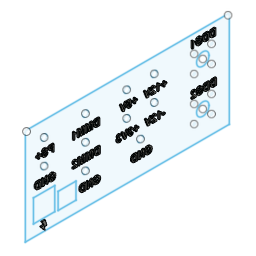
Schrift_Seitenteil_rechts (Autodesk Fusion 360 design; units mm, degrees)
Autodesk Fusion 360 part; units mm, degrees
(part 1 of 3)
sketch "Skizze1" plane through (-70, 0, 0) normal (-1, 0, 0) x (0, -1, 0)
  line L0 (-58.2934, 144.7089) -> (-56.3896, 144.7089)
  spline S0 degree 3 poles (-55.4941, 144.8148) (-55.624, 144.784) (-55.9182, 144.7143) (-56.2207, 144.7108) (-56.3896, 144.7089) knots 0 0 0 0 0.039934 0.090419 0.090419 0.090419 0.090419
  spline S1 degree 3 poles (-54.7832, 145.2147) (-54.8829, 145.1327) (-55.0958, 144.9574) (-55.3558, 144.8643) (-55.4941, 144.8148) knots 0 0 0 0 0.038436 0.082116 0.082116 0.082116 0.082116
  spline S2 degree 3 poles (-54.2466, 146.1) (-54.3131, 145.9292) (-54.4403, 145.6025) (-54.6724, 145.34) (-54.7832, 145.2147) knots 0 0 0 0 0.054482 0.104246 0.104246 0.104246 0.104246
  spline S3 degree 3 poles (-54.0928, 147.1664) (-54.0972, 146.9732) (-54.1056, 146.6113) (-54.2018, 146.2625) (-54.2466, 146.1) knots 0 0 0 0 0.057721 0.108107 0.108107 0.108107 0.108107
  spline S4 degree 3 poles (-54.2568, 148.3507) (-54.2091, 148.173) (-54.1049, 147.7854) (-54.097, 147.3838) (-54.0928, 147.1664) knots 0 0 0 0 0.055013 0.119956 0.119956 0.119956 0.119956
  spline S5 degree 3 poles (-54.7353, 149.1625) (-54.6361, 149.0437) (-54.4321, 148.7995) (-54.3163, 148.503) (-54.2568, 148.3507) knots 0 0 0 0 0.046108 0.094787 0.094787 0.094787 0.094787
  spline S6 degree 3 poles (-55.4907, 149.6239) (-55.3491, 149.5723) (-55.0663, 149.4692) (-54.8455, 149.2646) (-54.7353, 149.1625) knots 0 0 0 0 0.044725 0.089312 0.089312 0.089312 0.089312
  spline S7 degree 3 poles (-56.4443, 149.7196) (-56.2598, 149.7186) (-55.9386, 149.7169) (-55.6244, 149.6517) (-55.4907, 149.6239) knots 0 0 0 0 0.055167 0.096048 0.096048 0.096048 0.096048
  line L1 (-56.4443, 149.7196) -> (-58.2934, 149.7196)
  line L2 (-58.2934, 149.7196) -> (-58.2934, 144.7089)
  spline S8 degree 3 poles (-55.9966, 148.8241) (-56.101, 148.8379) (-56.3764, 148.8742) (-56.6545, 148.8728) (-56.8271, 148.872) knots 0 0 0 0 0.031565 0.083275 0.083275 0.083275 0.083275
  spline S9 degree 3 poles (-55.5283, 148.5883) (-55.5955, 148.642) (-55.7349, 148.7534) (-55.9073, 148.8) (-55.9966, 148.8241) knots 0 0 0 0 0.02553 0.052932 0.052932 0.052932 0.052932
  spline S10 degree 3 poles (-55.2412, 148.1029) (-55.2765, 148.1986) (-55.3427, 148.3782) (-55.4692, 148.5214) (-55.5283, 148.5883) knots 0 0 0 0 0.030297 0.056827 0.056827 0.056827 0.056827
  spline S11 degree 3 poles (-55.1387, 147.2108) (-55.1399, 147.3829) (-55.1421, 147.6843) (-55.2114, 147.9772) (-55.2412, 148.1029) knots 0 0 0 0 0.051419 0.090046 0.090046 0.090046 0.090046
  spline S12 degree 3 poles (-55.2412, 146.2931) (-55.2114, 146.4252) (-55.1433, 146.727) (-55.1403, 147.0367) (-55.1387, 147.2108) knots 0 0 0 0 0.040513 0.092572 0.092572 0.092572 0.092572
  spline S13 degree 3 poles (-55.5061, 145.8095) (-55.4529, 145.8719) (-55.3316, 146.0144) (-55.2737, 146.1929) (-55.2412, 146.2931) knots 0 0 0 0 0.024396 0.055616 0.055616 0.055616 0.055616
  spline S14 degree 3 poles (-55.9145, 145.601) (-55.8371, 145.624) (-55.688, 145.6684) (-55.5652, 145.7637) (-55.5061, 145.8095) knots 0 0 0 0 0.023993 0.046213 0.046213 0.046213 0.046213
  spline S15 degree 3 poles (-56.5264, 145.5531) (-56.4044, 145.5531) (-56.199, 145.553) (-55.9967, 145.5871) (-55.9145, 145.601) knots 0 0 0 0 0.036506 0.061461 0.061461 0.061461 0.061461
  line L3 (-56.5264, 145.5531) -> (-57.2817, 145.5531)
  line L4 (-57.2817, 145.5531) -> (-57.2817, 148.872)
  line L5 (-57.2817, 148.872) -> (-56.8271, 148.872)
  line L6 (-63.3486, 144.7089) -> (-61.4448, 144.7089)
  spline S16 degree 3 poles (-60.5493, 144.8148) (-60.6792, 144.784) (-60.9733, 144.7143) (-61.2759, 144.7108) (-61.4448, 144.7089) knots 0 0 0 0 0.039934 0.090419 0.090419 0.090419 0.090419
  spline S17 degree 3 poles (-59.8384, 145.2147) (-59.938, 145.1327) (-60.151, 144.9574) (-60.411, 144.8643) (-60.5493, 144.8148) knots 0 0 0 0 0.038436 0.082116 0.082116 0.082116 0.082116
  spline S18 degree 3 poles (-59.3017, 146.1) (-59.3683, 145.9292) (-59.4955, 145.6025) (-59.7276, 145.34) (-59.8384, 145.2147) knots 0 0 0 0 0.054482 0.104246 0.104246 0.104246 0.104246
  spline S19 degree 3 poles (-59.1479, 147.1664) (-59.1524, 146.9732) (-59.1608, 146.6113) (-59.2569, 146.2625) (-59.3017, 146.1) knots 0 0 0 0 0.057721 0.108107 0.108107 0.108107 0.108107
  spline S20 degree 3 poles (-59.312, 148.3507) (-59.2642, 148.173) (-59.1601, 147.7854) (-59.1522, 147.3838) (-59.1479, 147.1664) knots 0 0 0 0 0.055013 0.119956 0.119956 0.119956 0.119956
  spline S21 degree 3 poles (-59.7905, 149.1625) (-59.6913, 149.0437) (-59.4872, 148.7995) (-59.3715, 148.503) (-59.312, 148.3507) knots 0 0 0 0 0.046108 0.094787 0.094787 0.094787 0.094787
  spline S22 degree 3 poles (-60.5459, 149.6239) (-60.4043, 149.5723) (-60.1215, 149.4692) (-59.9007, 149.2646) (-59.7905, 149.1625) knots 0 0 0 0 0.044725 0.089312 0.089312 0.089312 0.089312
  spline S23 degree 3 poles (-61.4995, 149.7196) (-61.315, 149.7186) (-60.9938, 149.7169) (-60.6796, 149.6517) (-60.5459, 149.6239) knots 0 0 0 0 0.055167 0.096048 0.096048 0.096048 0.096048
  line L7 (-61.4995, 149.7196) -> (-63.3486, 149.7196)
  line L8 (-63.3486, 149.7196) -> (-63.3486, 144.7089)
  spline S24 degree 3 poles (-61.0517, 148.8241) (-61.1562, 148.8379) (-61.4316, 148.8742) (-61.7097, 148.8728) (-61.8823, 148.872) knots 0 0 0 0 0.031565 0.083275 0.083275 0.083275 0.083275
  spline S25 degree 3 poles (-60.5835, 148.5883) (-60.6507, 148.642) (-60.7901, 148.7534) (-60.9625, 148.8) (-61.0517, 148.8241) knots 0 0 0 0 0.02553 0.052932 0.052932 0.052932 0.052932
  spline S26 degree 3 poles (-60.2964, 148.1029) (-60.3317, 148.1986) (-60.3979, 148.3782) (-60.5244, 148.5214) (-60.5835, 148.5883) knots 0 0 0 0 0.030297 0.056827 0.056827 0.056827 0.056827
  spline S27 degree 3 poles (-60.1938, 147.2108) (-60.1951, 147.3829) (-60.1973, 147.6843) (-60.2666, 147.9772) (-60.2964, 148.1029) knots 0 0 0 0 0.051419 0.090046 0.090046 0.090046 0.090046
  spline S28 degree 3 poles (-60.2964, 146.2931) (-60.2666, 146.4252) (-60.1985, 146.727) (-60.1955, 147.0367) (-60.1938, 147.2108) knots 0 0 0 0 0.040513 0.092572 0.092572 0.092572 0.092572
  spline S29 degree 3 poles (-60.5613, 145.8095) (-60.5081, 145.8719) (-60.3868, 146.0144) (-60.3289, 146.1929) (-60.2964, 146.2931) knots 0 0 0 0 0.024396 0.055616 0.055616 0.055616 0.055616
  spline S30 degree 3 poles (-60.9697, 145.601) (-60.8923, 145.624) (-60.7432, 145.6684) (-60.6203, 145.7637) (-60.5613, 145.8095) knots 0 0 0 0 0.023993 0.046213 0.046213 0.046213 0.046213
  spline S31 degree 3 poles (-61.5815, 145.5531) (-61.4596, 145.5531) (-61.2542, 145.553) (-61.0519, 145.5871) (-60.9697, 145.601) knots 0 0 0 0 0.036506 0.061461 0.061461 0.061461 0.061461
  line L9 (-61.5815, 145.5531) -> (-62.3369, 145.5531)
  line L10 (-62.3369, 145.5531) -> (-62.3369, 148.872)
  line L11 (-62.3369, 148.872) -> (-61.8823, 148.872)
  spline S32 degree 3 poles (-51.4233, 144.62) (-51.7117, 144.6304) (-52.2389, 144.6493) (-52.6821, 144.9314) (-52.8828, 145.0592) knots 0 0 0 0 0.084711 0.154875 0.154875 0.154875 0.154875
  spline S33 degree 3 poles (-50.333, 144.8029) (-50.4955, 144.7496) (-50.8492, 144.6337) (-51.2218, 144.6248) (-51.4233, 144.62) knots 0 0 0 0 0.051012 0.111086 0.111086 0.111086 0.111086
  spline S34 degree 3 poles (-49.6562, 145.3617) (-49.7454, 145.2439) (-49.9268, 145.0044) (-50.1961, 144.8708) (-50.333, 144.8029) knots 0 0 0 0 0.043681 0.088839 0.088839 0.088839 0.088839
  spline S35 degree 3 poles (-49.417, 146.1683) (-49.4273, 146.0265) (-49.4482, 145.7402) (-49.5865, 145.4886) (-49.6562, 145.3617) knots 0 0 0 0 0.042126 0.085024 0.085024 0.085024 0.085024
  spline S36 degree 3 poles (-49.6169, 146.9664) (-49.5587, 146.8482) (-49.4348, 146.597) (-49.4232, 146.3167) (-49.417, 146.1683) knots 0 0 0 0 0.039093 0.083085 0.083085 0.083085 0.083085
  spline S37 degree 3 poles (-50.1706, 147.4757) (-50.0596, 147.4087) (-49.8405, 147.2764) (-49.6908, 147.0688) (-49.6169, 146.9664) knots 0 0 0 0 0.038473 0.075924 0.075924 0.075924 0.075924
  spline S38 degree 3 poles (-51.2627, 147.8363) (-51.0462, 147.7843) (-50.6719, 147.6945) (-50.3193, 147.5406) (-50.1706, 147.4757) knots 0 0 0 0 0.066618 0.115197 0.115197 0.115197 0.115197
  spline S39 degree 3 poles (-52.1924, 148.1713) (-52.0845, 148.1126) (-51.7928, 147.9541) (-51.4676, 147.8818) (-51.2627, 147.8363) knots 0 0 0 0 0.036685 0.099222 0.099222 0.099222 0.099222
  spline S40 degree 3 poles (-52.3428, 148.4755) (-52.3358, 148.4178) (-52.3215, 148.299) (-52.2362, 148.2147) (-52.1924, 148.1713) knots 0 0 0 0 0.016915 0.034837 0.034837 0.034837 0.034837
  spline S41 degree 3 poles (-52.1821, 148.7865) (-52.229, 148.7447) (-52.3222, 148.6614) (-52.3359, 148.5372) (-52.3428, 148.4755) knots 0 0 0 0 0.018159 0.036131 0.036131 0.036131 0.036131
  spline S42 degree 3 poles (-51.4917, 148.9677) (-51.6257, 148.9634) (-51.8706, 148.9557) (-52.0851, 148.8392) (-52.1821, 148.7865) knots 0 0 0 0 0.039567 0.07226 0.07226 0.07226 0.07226
  spline S43 degree 3 poles (-50.8508, 148.7985) (-50.9379, 148.8476) (-51.1357, 148.9594) (-51.3639, 148.9647) (-51.4917, 148.9677) knots 0 0 0 0 0.029564 0.067187 0.067187 0.067187 0.067187
  spline S44 degree 3 poles (-50.5723, 148.243) (-50.5959, 148.3591) (-50.639, 148.5704) (-50.785, 148.7276) (-50.8508, 148.7985) knots 0 0 0 0 0.034732 0.063204 0.063204 0.063204 0.063204
  line L12 (-50.5723, 148.243) -> (-49.5605, 148.2875)
  spline S45 degree 3 poles (-50.0613, 149.3915) (-49.9211, 149.2393) (-49.6335, 148.9268) (-49.5853, 148.5042) (-49.5605, 148.2875) knots 0 0 0 0 0.060438 0.124056 0.124056 0.124056 0.124056
  spline S46 degree 3 poles (-51.4814, 149.8051) (-51.1977, 149.7967) (-50.6859, 149.7816) (-50.2538, 149.5117) (-50.0613, 149.3915) knots 0 0 0 0 0.083316 0.150278 0.150278 0.150278 0.150278
  spline S47 degree 3 poles (-52.4675, 149.6307) (-52.3186, 149.6815) (-51.9992, 149.7904) (-51.6616, 149.8) (-51.4814, 149.8051) knots 0 0 0 0 0.046932 0.100643 0.100643 0.100643 0.100643
  spline S48 degree 3 poles (-53.093, 149.1232) (-53.0108, 149.2284) (-52.8414, 149.4453) (-52.5946, 149.5677) (-52.4675, 149.6307) knots 0 0 0 0 0.039537 0.081471 0.081471 0.081471 0.081471
  spline S49 degree 3 poles (-53.31, 148.4071) (-53.3006, 148.5332) (-53.2816, 148.788) (-53.1563, 149.0107) (-53.093, 149.1232) knots 0 0 0 0 0.037438 0.075643 0.075643 0.075643 0.075643
  spline S50 degree 3 poles (-52.8486, 147.3988) (-52.9832, 147.543) (-53.2492, 147.8281) (-53.2899, 148.2156) (-53.31, 148.4071) knots 0 0 0 0 0.057473 0.113615 0.113615 0.113615 0.113615
  spline S51 degree 3 poles (-51.707, 146.9032) (-51.9444, 146.9635) (-52.353, 147.0673) (-52.7023, 147.3009) (-52.8486, 147.3988) knots 0 0 0 0 0.072771 0.125248 0.125248 0.125248 0.125248
  spline S52 degree 3 poles (-50.897, 146.6845) (-50.9939, 146.7135) (-51.2619, 146.7939) (-51.5336, 146.8606) (-51.707, 146.9032) knots 0 0 0 0 0.030365 0.083919 0.083919 0.083919 0.083919
  spline S53 degree 3 poles (-50.5329, 146.4674) (-50.5789, 146.5092) (-50.6851, 146.6059) (-50.8202, 146.656) (-50.897, 146.6845) knots 0 0 0 0 0.018463 0.042727 0.042727 0.042727 0.042727
  spline S54 degree 3 poles (-50.4287, 146.1649) (-50.4326, 146.2214) (-50.4402, 146.3317) (-50.5025, 146.4229) (-50.5329, 146.4674) knots 0 0 0 0 0.016654 0.032515 0.032515 0.032515 0.032515
  spline S55 degree 3 poles (-50.6765, 145.6813) (-50.6043, 145.7509) (-50.4659, 145.8843) (-50.4407, 146.0742) (-50.4287, 146.1649) knots 0 0 0 0 0.02913 0.055793 0.055793 0.055793 0.055793
  spline S56 degree 3 poles (-51.4131, 145.4745) (-51.2662, 145.4785) (-51.0021, 145.4858) (-50.7766, 145.6212) (-50.6765, 145.6813) knots 0 0 0 0 0.043163 0.077652 0.077652 0.077652 0.077652
  spline S57 degree 3 poles (-52.1462, 145.7069) (-52.043, 145.6392) (-51.8212, 145.4937) (-51.5553, 145.4812) (-51.4131, 145.4745) knots 0 0 0 0 0.036365 0.078171 0.078171 0.078171 0.078171
  spline S58 degree 3 poles (-52.5068, 146.4349) (-52.4745, 146.2852) (-52.4153, 146.0111) (-52.2302, 145.8019) (-52.1462, 145.7069) knots 0 0 0 0 0.045039 0.082457 0.082457 0.082457 0.082457
  line L13 (-52.5068, 146.4349) -> (-53.4912, 146.3392)
  spline S59 degree 3 poles (-52.8828, 145.0592) (-53.0363, 145.2303) (-53.364, 145.5957) (-53.447, 146.0811) (-53.4912, 146.3392) knots 0 0 0 0 0.067573 0.144312 0.144312 0.144312 0.144312
  line L14 (-46.3203, 149.7401) -> (-47.0996, 149.7401)
  spline S60 degree 3 poles (-47.7046, 148.9386) (-47.5703, 149.0549) (-47.3111, 149.2791) (-47.1684, 149.5903) (-47.0996, 149.7401) knots 0 0 0 0 0.052597 0.101463 0.101463 0.101463 0.101463
  spline S61 degree 3 poles (-48.5215, 148.4721) (-48.388, 148.5266) (-48.0955, 148.6461) (-47.8423, 148.8356) (-47.7046, 148.9386) knots 0 0 0 0 0.043078 0.094413 0.094413 0.094413 0.094413
  line L15 (-48.5215, 148.4721) -> (-48.5215, 147.6005)
  spline S62 degree 3 poles (-47.2808, 148.3285) (-47.4653, 148.1747) (-47.8387, 147.8636) (-48.2922, 147.6888) (-48.5215, 147.6005) knots 0 0 0 0 0.071555 0.144721 0.144721 0.144721 0.144721
  line L16 (-47.2808, 148.3285) -> (-47.2808, 144.7089)
  line L17 (-47.2808, 144.7089) -> (-46.3203, 144.7089)
  line L18 (-46.3203, 144.7089) -> (-46.3203, 149.7401)
  line L19 (-63.8491, 113.2089) -> (-61.9453, 113.2089)
  spline S63 degree 3 poles (-61.0498, 113.3148) (-61.1797, 113.284) (-61.4739, 113.2143) (-61.7764, 113.2108) (-61.9453, 113.2089) knots 0 0 0 0 0.039934 0.090419 0.090419 0.090419 0.090419
  spline S64 degree 3 poles (-60.3389, 113.7147) (-60.4386, 113.6327) (-60.6515, 113.4574) (-60.9115, 113.3643) (-61.0498, 113.3148) knots 0 0 0 0 0.038436 0.082116 0.082116 0.082116 0.082116
  spline S65 degree 3 poles (-59.8023, 114.6) (-59.8688, 114.4292) (-59.996, 114.1025) (-60.2281, 113.84) (-60.3389, 113.7147) knots 0 0 0 0 0.054482 0.104246 0.104246 0.104246 0.104246
  spline S66 degree 3 poles (-59.6485, 115.6664) (-59.6529, 115.4732) (-59.6613, 115.1113) (-59.7575, 114.7625) (-59.8023, 114.6) knots 0 0 0 0 0.057721 0.108107 0.108107 0.108107 0.108107
  spline S67 degree 3 poles (-59.8125, 116.8507) (-59.7647, 116.673) (-59.6606, 116.2854) (-59.6527, 115.8838) (-59.6485, 115.6664) knots 0 0 0 0 0.055013 0.119956 0.119956 0.119956 0.119956
  spline S68 degree 3 poles (-60.291, 117.6625) (-60.1918, 117.5437) (-59.9878, 117.2995) (-59.872, 117.003) (-59.8125, 116.8507) knots 0 0 0 0 0.046108 0.094787 0.094787 0.094787 0.094787
  spline S69 degree 3 poles (-61.0464, 118.1239) (-60.9048, 118.0723) (-60.622, 117.9692) (-60.4012, 117.7646) (-60.291, 117.6625) knots 0 0 0 0 0.044725 0.089312 0.089312 0.089312 0.089312
  spline S70 degree 3 poles (-62, 118.2196) (-61.8155, 118.2186) (-61.4943, 118.2169) (-61.1801, 118.1517) (-61.0464, 118.1239) knots 0 0 0 0 0.055167 0.096048 0.096048 0.096048 0.096048
  line L20 (-62, 118.2196) -> (-63.8491, 118.2196)
  line L21 (-63.8491, 118.2196) -> (-63.8491, 113.2089)
  spline S71 degree 3 poles (-61.5523, 117.3241) (-61.6567, 117.3379) (-61.9321, 117.3742) (-62.2102, 117.3728) (-62.3828, 117.372) knots 0 0 0 0 0.031565 0.083275 0.083275 0.083275 0.083275
  spline S72 degree 3 poles (-61.084, 117.0883) (-61.1512, 117.142) (-61.2906, 117.2534) (-61.463, 117.3) (-61.5523, 117.3241) knots 0 0 0 0 0.02553 0.052932 0.052932 0.052932 0.052932
  spline S73 degree 3 poles (-60.7969, 116.6029) (-60.8322, 116.6986) (-60.8984, 116.8782) (-61.0249, 117.0214) (-61.084, 117.0883) knots 0 0 0 0 0.030297 0.056827 0.056827 0.056827 0.056827
  spline S74 degree 3 poles (-60.6944, 115.7108) (-60.6956, 115.8829) (-60.6978, 116.1843) (-60.7671, 116.4772) (-60.7969, 116.6029) knots 0 0 0 0 0.051419 0.090046 0.090046 0.090046 0.090046
  spline S75 degree 3 poles (-60.7969, 114.7931) (-60.7671, 114.9252) (-60.699, 115.227) (-60.696, 115.5367) (-60.6944, 115.7108) knots 0 0 0 0 0.040513 0.092572 0.092572 0.092572 0.092572
  spline S76 degree 3 poles (-61.0618, 114.3095) (-61.0086, 114.3719) (-60.8873, 114.5144) (-60.8294, 114.6929) (-60.7969, 114.7931) knots 0 0 0 0 0.024396 0.055616 0.055616 0.055616 0.055616
  spline S77 degree 3 poles (-61.4702, 114.101) (-61.3928, 114.124) (-61.2437, 114.1684) (-61.1209, 114.2637) (-61.0618, 114.3095) knots 0 0 0 0 0.023993 0.046213 0.046213 0.046213 0.046213
  spline S78 degree 3 poles (-62.082, 114.0531) (-61.9601, 114.0531) (-61.7547, 114.053) (-61.5524, 114.0871) (-61.4702, 114.101) knots 0 0 0 0 0.036506 0.061461 0.061461 0.061461 0.061461
  line L22 (-62.082, 114.0531) -> (-62.8374, 114.0531)
  line L23 (-62.8374, 114.0531) -> (-62.8374, 117.372)
  line L24 (-62.8374, 117.372) -> (-62.3828, 117.372)
  line L25 (-58.794, 113.2089) -> (-56.8902, 113.2089)
  spline S79 degree 3 poles (-55.9946, 113.3148) (-56.1245, 113.284) (-56.4187, 113.2143) (-56.7212, 113.2108) (-56.8902, 113.2089) knots 0 0 0 0 0.039934 0.090419 0.090419 0.090419 0.090419
  spline S80 degree 3 poles (-55.2837, 113.7147) (-55.3834, 113.6327) (-55.5963, 113.4574) (-55.8563, 113.3643) (-55.9946, 113.3148) knots 0 0 0 0 0.038436 0.082116 0.082116 0.082116 0.082116
  spline S81 degree 3 poles (-54.7471, 114.6) (-54.8136, 114.4292) (-54.9408, 114.1025) (-55.1729, 113.84) (-55.2837, 113.7147) knots 0 0 0 0 0.054482 0.104246 0.104246 0.104246 0.104246
  spline S82 degree 3 poles (-54.5933, 115.6664) (-54.5978, 115.4732) (-54.6061, 115.1113) (-54.7023, 114.7625) (-54.7471, 114.6) knots 0 0 0 0 0.057721 0.108107 0.108107 0.108107 0.108107
  spline S83 degree 3 poles (-54.7573, 116.8507) (-54.7096, 116.673) (-54.6054, 116.2854) (-54.5975, 115.8838) (-54.5933, 115.6664) knots 0 0 0 0 0.055013 0.119956 0.119956 0.119956 0.119956
  spline S84 degree 3 poles (-55.2359, 117.6625) (-55.1366, 117.5437) (-54.9326, 117.2995) (-54.8168, 117.003) (-54.7573, 116.8507) knots 0 0 0 0 0.046108 0.094787 0.094787 0.094787 0.094787
  spline S85 degree 3 poles (-55.9912, 118.1239) (-55.8496, 118.0723) (-55.5668, 117.9692) (-55.3461, 117.7646) (-55.2359, 117.6625) knots 0 0 0 0 0.044725 0.089312 0.089312 0.089312 0.089312
  spline S86 degree 3 poles (-56.9448, 118.2196) (-56.7604, 118.2186) (-56.4392, 118.2169) (-56.125, 118.1517) (-55.9912, 118.1239) knots 0 0 0 0 0.055167 0.096048 0.096048 0.096048 0.096048
  line L26 (-56.9448, 118.2196) -> (-58.794, 118.2196)
  line L27 (-58.794, 118.2196) -> (-58.794, 113.2089)
  spline S87 degree 3 poles (-56.4971, 117.3241) (-56.6015, 117.3379) (-56.877, 117.3742) (-57.155, 117.3728) (-57.3277, 117.372) knots 0 0 0 0 0.031565 0.083275 0.083275 0.083275 0.083275
  spline S88 degree 3 poles (-56.0288, 117.0883) (-56.096, 117.142) (-56.2354, 117.2534) (-56.4078, 117.3) (-56.4971, 117.3241) knots 0 0 0 0 0.02553 0.052932 0.052932 0.052932 0.052932
  spline S89 degree 3 poles (-55.7417, 116.6029) (-55.777, 116.6986) (-55.8432, 116.8782) (-55.9698, 117.0214) (-56.0288, 117.0883) knots 0 0 0 0 0.030297 0.056827 0.056827 0.056827 0.056827
  spline S90 degree 3 poles (-55.6392, 115.7108) (-55.6404, 115.8829) (-55.6426, 116.1843) (-55.712, 116.4772) (-55.7417, 116.6029) knots 0 0 0 0 0.051419 0.090046 0.090046 0.090046 0.090046
  spline S91 degree 3 poles (-55.7417, 114.7931) (-55.7119, 114.9252) (-55.6439, 115.227) (-55.6409, 115.5367) (-55.6392, 115.7108) knots 0 0 0 0 0.040513 0.092572 0.092572 0.092572 0.092572
  spline S92 degree 3 poles (-56.0066, 114.3095) (-55.9534, 114.3719) (-55.8321, 114.5144) (-55.7742, 114.6929) (-55.7417, 114.7931) knots 0 0 0 0 0.024396 0.055616 0.055616 0.055616 0.055616
  spline S93 degree 3 poles (-56.4151, 114.101) (-56.3376, 114.124) (-56.1885, 114.1684) (-56.0657, 114.2637) (-56.0066, 114.3095) knots 0 0 0 0 0.023993 0.046213 0.046213 0.046213 0.046213
  spline S94 degree 3 poles (-57.0269, 114.0531) (-56.9049, 114.0531) (-56.6995, 114.053) (-56.4972, 114.0871) (-56.4151, 114.101) knots 0 0 0 0 0.036506 0.061461 0.061461 0.061461 0.061461
  line L28 (-57.0269, 114.0531) -> (-57.7822, 114.0531)
  line L29 (-57.7822, 114.0531) -> (-57.7822, 117.372)
  line L30 (-57.7822, 117.372) -> (-57.3277, 117.372)
  spline S95 degree 3 poles (-51.9238, 113.12) (-52.2122, 113.1304) (-52.7395, 113.1493) (-53.1826, 113.4314) (-53.3833, 113.5592) knots 0 0 0 0 0.084711 0.154875 0.154875 0.154875 0.154875
  spline S96 degree 3 poles (-50.8335, 113.3029) (-50.996, 113.2496) (-51.3497, 113.1337) (-51.7223, 113.1248) (-51.9238, 113.12) knots 0 0 0 0 0.051012 0.111086 0.111086 0.111086 0.111086
  spline S97 degree 3 poles (-50.1568, 113.8617) (-50.2459, 113.7439) (-50.4273, 113.5044) (-50.6966, 113.3708) (-50.8335, 113.3029) knots 0 0 0 0 0.043681 0.088839 0.088839 0.088839 0.088839
  spline S98 degree 3 poles (-49.9175, 114.6683) (-49.9278, 114.5265) (-49.9487, 114.2402) (-50.087, 113.9886) (-50.1568, 113.8617) knots 0 0 0 0 0.042126 0.085024 0.085024 0.085024 0.085024
  spline S99 degree 3 poles (-50.1174, 115.4664) (-50.0592, 115.3482) (-49.9354, 115.097) (-49.9237, 114.8167) (-49.9175, 114.6683) knots 0 0 0 0 0.039093 0.083085 0.083085 0.083085 0.083085
  spline S100 degree 3 poles (-50.6712, 115.9757) (-50.5601, 115.9087) (-50.341, 115.7764) (-50.1913, 115.5688) (-50.1174, 115.4664) knots 0 0 0 0 0.038473 0.075924 0.075924 0.075924 0.075924
  spline S101 degree 3 poles (-51.7632, 116.3363) (-51.5467, 116.2843) (-51.1724, 116.1945) (-50.8198, 116.0406) (-50.6712, 115.9757) knots 0 0 0 0 0.066618 0.115197 0.115197 0.115197 0.115197
  spline S102 degree 3 poles (-52.6929, 116.6713) (-52.585, 116.6126) (-52.2933, 116.4541) (-51.9682, 116.3818) (-51.7632, 116.3363) knots 0 0 0 0 0.036685 0.099222 0.099222 0.099222 0.099222
  spline S103 degree 3 poles (-52.8433, 116.9755) (-52.8363, 116.9178) (-52.822, 116.799) (-52.7367, 116.7147) (-52.6929, 116.6713) knots 0 0 0 0 0.016915 0.034837 0.034837 0.034837 0.034837
  spline S104 degree 3 poles (-52.6826, 117.2865) (-52.7295, 117.2447) (-52.8227, 117.1614) (-52.8364, 117.0372) (-52.8433, 116.9755) knots 0 0 0 0 0.018159 0.036131 0.036131 0.036131 0.036131
  spline S105 degree 3 poles (-51.9922, 117.4677) (-52.1263, 117.4634) (-52.3711, 117.4557) (-52.5856, 117.3392) (-52.6826, 117.2865) knots 0 0 0 0 0.039567 0.07226 0.07226 0.07226 0.07226
  spline S106 degree 3 poles (-51.3513, 117.2985) (-51.4384, 117.3476) (-51.6362, 117.4594) (-51.8644, 117.4647) (-51.9922, 117.4677) knots 0 0 0 0 0.029564 0.067187 0.067187 0.067187 0.067187
  spline S107 degree 3 poles (-51.0728, 116.743) (-51.0964, 116.8591) (-51.1395, 117.0704) (-51.2856, 117.2276) (-51.3513, 117.2985) knots 0 0 0 0 0.034732 0.063204 0.063204 0.063204 0.063204
  line L31 (-51.0728, 116.743) -> (-50.061, 116.7875)
  spline S108 degree 3 poles (-50.5618, 117.8915) (-50.4216, 117.7393) (-50.134, 117.4268) (-50.0858, 117.0042) (-50.061, 116.7875) knots 0 0 0 0 0.060438 0.124056 0.124056 0.124056 0.124056
  spline S109 degree 3 poles (-51.9819, 118.3051) (-51.6982, 118.2967) (-51.1864, 118.2816) (-50.7543, 118.0117) (-50.5618, 117.8915) knots 0 0 0 0 0.083316 0.150278 0.150278 0.150278 0.150278
  spline S110 degree 3 poles (-52.968, 118.1307) (-52.8191, 118.1815) (-52.4997, 118.2904) (-52.1621, 118.3) (-51.9819, 118.3051) knots 0 0 0 0 0.046932 0.100643 0.100643 0.100643 0.100643
  spline S111 degree 3 poles (-53.5935, 117.6232) (-53.5113, 117.7284) (-53.3419, 117.9453) (-53.0951, 118.0677) (-52.968, 118.1307) knots 0 0 0 0 0.039537 0.081471 0.081471 0.081471 0.081471
  spline S112 degree 3 poles (-53.8106, 116.9071) (-53.8012, 117.0332) (-53.7822, 117.288) (-53.6568, 117.5107) (-53.5935, 117.6232) knots 0 0 0 0 0.037438 0.075643 0.075643 0.075643 0.075643
  spline S113 degree 3 poles (-53.3491, 115.8988) (-53.4837, 116.043) (-53.7497, 116.3281) (-53.7904, 116.7156) (-53.8106, 116.9071) knots 0 0 0 0 0.057473 0.113615 0.113615 0.113615 0.113615
  spline S114 degree 3 poles (-52.2075, 115.4032) (-52.4449, 115.4635) (-52.8535, 115.5673) (-53.2028, 115.8009) (-53.3491, 115.8988) knots 0 0 0 0 0.072771 0.125248 0.125248 0.125248 0.125248
  spline S115 degree 3 poles (-51.3975, 115.1845) (-51.4944, 115.2135) (-51.7624, 115.2939) (-52.0341, 115.3606) (-52.2075, 115.4032) knots 0 0 0 0 0.030365 0.083919 0.083919 0.083919 0.083919
  spline S116 degree 3 poles (-51.0335, 114.9674) (-51.0794, 115.0092) (-51.1856, 115.1059) (-51.3207, 115.156) (-51.3975, 115.1845) knots 0 0 0 0 0.018463 0.042727 0.042727 0.042727 0.042727
  spline S117 degree 3 poles (-50.9292, 114.6649) (-50.9331, 114.7214) (-50.9407, 114.8317) (-51.0031, 114.9229) (-51.0335, 114.9674) knots 0 0 0 0 0.016654 0.032515 0.032515 0.032515 0.032515
  spline S118 degree 3 poles (-51.177, 114.1813) (-51.1048, 114.2509) (-50.9664, 114.3843) (-50.9412, 114.5742) (-50.9292, 114.6649) knots 0 0 0 0 0.02913 0.055793 0.055793 0.055793 0.055793
  spline S119 degree 3 poles (-51.9136, 113.9745) (-51.7668, 113.9785) (-51.5026, 113.9858) (-51.2772, 114.1212) (-51.177, 114.1813) knots 0 0 0 0 0.043163 0.077652 0.077652 0.077652 0.077652
  spline S120 degree 3 poles (-52.6467, 114.2069) (-52.5435, 114.1392) (-52.3217, 113.9937) (-52.0558, 113.9812) (-51.9136, 113.9745) knots 0 0 0 0 0.036365 0.078171 0.078171 0.078171 0.078171
  spline S121 degree 3 poles (-53.0073, 114.9349) (-52.975, 114.7852) (-52.9158, 114.5111) (-52.7307, 114.3019) (-52.6467, 114.2069) knots 0 0 0 0 0.045039 0.082457 0.082457 0.082457 0.082457
  line L32 (-53.0073, 114.9349) -> (-53.9917, 114.8392)
  spline S122 degree 3 poles (-53.3833, 113.5592) (-53.5368, 113.7303) (-53.8645, 114.0957) (-53.9476, 114.5811) (-53.9917, 114.8392) knots 0 0 0 0 0.067573 0.144312 0.144312 0.144312 0.144312
  spline S123 degree 3 poles (-47.7454, 114.3676) (-47.7832, 114.3235) (-47.8553, 114.2394) (-47.914, 114.1456) (-47.9419, 114.101) knots 0 0 0 0 0.017402 0.033163 0.033163 0.033163 0.033163
  spline S124 degree 3 poles (-47.1694, 114.9213) (-47.2947, 114.8071) (-47.4916, 114.6277) (-47.6776, 114.437) (-47.7454, 114.3676) knots 0 0 0 0 0.050814 0.079907 0.079907 0.079907 0.079907
  spline S125 degree 3 poles (-46.5405, 115.5604) (-46.6207, 115.4689) (-46.8179, 115.2437) (-47.0385, 115.0414) (-47.1694, 114.9213) knots 0 0 0 0 0.036482 0.089726 0.089726 0.089726 0.089726
  spline S126 degree 3 poles (-46.156, 116.2013) (-46.2049, 116.0949) (-46.3096, 115.8673) (-46.4603, 115.6671) (-46.5405, 115.5604) knots 0 0 0 0 0.035023 0.074928 0.074928 0.074928 0.074928
  spline S127 degree 3 poles (-46.0347, 116.8456) (-46.0396, 116.7345) (-46.0493, 116.5139) (-46.1206, 116.305) (-46.156, 116.2013) knots 0 0 0 0 0.033165 0.06586 0.06586 0.06586 0.06586
  spline S128 degree 3 poles (-46.4585, 117.8402) (-46.3349, 117.6982) (-46.0862, 117.4126) (-46.0519, 117.0353) (-46.0347, 116.8456) knots 0 0 0 0 0.054981 0.110602 0.110602 0.110602 0.110602
  spline S129 degree 3 poles (-47.624, 118.2401) (-47.3956, 118.2284) (-46.9672, 118.2064) (-46.6204, 117.9567) (-46.4585, 117.8402) knots 0 0 0 0 0.066974 0.125562 0.125562 0.125562 0.125562
  spline S130 degree 3 poles (-48.752, 117.8949) (-48.5873, 117.9955) (-48.2416, 118.2068) (-47.8363, 118.2287) (-47.624, 118.2401) knots 0 0 0 0 0.056979 0.119613 0.119613 0.119613 0.119613
  spline S131 degree 3 poles (-49.2886, 116.7567) (-49.2532, 116.9954) (-49.1885, 117.4315) (-48.888, 117.7505) (-48.752, 117.8949) knots 0 0 0 0 0.070363 0.128535 0.128535 0.128535 0.128535
  line L33 (-49.2886, 116.7567) -> (-48.3316, 116.661)
  spline S132 degree 3 poles (-48.1265, 117.2626) (-48.1797, 117.1847) (-48.303, 117.0043) (-48.3212, 116.7854) (-48.3316, 116.661) knots 0 0 0 0 0.027875 0.064515 0.064515 0.064515 0.064515
  spline S133 degree 3 poles (-47.648, 117.4437) (-47.7415, 117.4377) (-47.9201, 117.4263) (-48.0599, 117.3154) (-48.1265, 117.2626) knots 0 0 0 0 0.027379 0.052265 0.052265 0.052265 0.052265
  spline S134 degree 3 poles (-47.1712, 117.2711) (-47.237, 117.3214) (-47.3772, 117.4286) (-47.5541, 117.4385) (-47.648, 117.4437) knots 0 0 0 0 0.024288 0.051759 0.051759 0.051759 0.051759
  spline S135 degree 3 poles (-46.9985, 116.7772) (-47.0033, 116.8755) (-47.012, 117.058) (-47.1209, 117.2038) (-47.1712, 117.2711) knots 0 0 0 0 0.028738 0.053388 0.053388 0.053388 0.053388
  spline S136 degree 3 poles (-47.1968, 116.1893) (-47.139, 116.2852) (-47.0295, 116.4669) (-47.0085, 116.6777) (-46.9985, 116.7772) knots 0 0 0 0 0.033093 0.062734 0.062734 0.062734 0.062734
  spline S137 degree 3 poles (-47.9932, 115.369) (-47.8138, 115.5337) (-47.5325, 115.7921) (-47.2861, 116.0836) (-47.1968, 116.1893) knots 0 0 0 0 0.072938 0.114424 0.114424 0.114424 0.114424
  spline S138 degree 3 poles (-49.0733, 114.1676) (-48.942, 114.347) (-48.6228, 114.7834) (-48.2265, 115.152) (-47.9932, 115.369) knots 0 0 0 0 0.066554 0.16187 0.16187 0.16187 0.16187
  spline S139 degree 3 poles (-49.4014, 113.2089) (-49.3736, 113.376) (-49.3174, 113.7138) (-49.1552, 114.0153) (-49.0733, 114.1676) knots 0 0 0 0 0.050461 0.101951 0.101951 0.101951 0.101951
  line L34 (-49.4014, 113.2089) -> (-46.0347, 113.2089)
  line L35 (-46.0347, 113.2089) -> (-46.0347, 114.101)
  line L36 (-46.0347, 114.101) -> (-47.9419, 114.101)
  line L37 (4.1011, 130.5054) -> (5.8956, 135.5162)
  line L38 (5.8956, 135.5162) -> (4.8223, 135.5162)
  line L39 (4.8223, 135.5162) -> (3.5953, 131.8077)
  line L40 (3.5953, 131.8077) -> (2.3272, 135.5162)
  line L41 (2.3272, 135.5162) -> (1.23, 135.5162)
  line L42 (1.23, 135.5162) -> (3.0211, 130.5054)
  line L43 (3.0211, 130.5054) -> (4.1011, 130.5054)
  spline S140 degree 3 poles (-0.6943, 130.42) (-0.9106, 130.4321) (-1.3222, 130.455) (-1.6637, 130.684) (-1.8256, 130.7926) knots 0 0 0 0 0.063661 0.121078 0.121078 0.121078 0.121078
  spline S141 degree 3 poles (0.6627, 131.0831) (0.4818, 130.8897) (0.1142, 130.4968) (-0.422, 130.4459) (-0.6943, 130.42) knots 0 0 0 0 0.076677 0.155765 0.155765 0.155765 0.155765
  spline S142 degree 3 poles (1.0216, 132.1871) (1.007, 131.987) (0.9781, 131.5894) (0.7673, 131.2511) (0.6627, 131.0831) knots 0 0 0 0 0.059216 0.117652 0.117652 0.117652 0.117652
  spline S143 degree 3 poles (0.5772, 133.3936) (0.7068, 133.2226) (0.9766, 132.8663) (1.0062, 132.4194) (1.0216, 132.1871) knots 0 0 0 0 0.06295 0.13111 0.13111 0.13111 0.13111
  spline S144 degree 3 poles (-0.5063, 133.8585) (-0.3012, 133.839) (0.1096, 133.7999) (0.4212, 133.5292) (0.5772, 133.3936) knots 0 0 0 0 0.060178 0.120563 0.120563 0.120563 0.120563
  spline S145 degree 3 poles (-1.1625, 133.6978) (-1.0559, 133.7447) (-0.8465, 133.8367) (-0.6183, 133.8513) (-0.5063, 133.8585) knots 0 0 0 0 0.034634 0.068031 0.068031 0.068031 0.068031
  line L44 (-1.1625, 133.6978) -> (-1.0121, 134.5489)
  line L45 (-1.0121, 134.5489) -> (0.7994, 134.5489)
  line L46 (0.7994, 134.5489) -> (0.7994, 135.4478)
  line L47 (0.7994, 135.4478) -> (-1.7402, 135.4478)
  line L48 (-1.7402, 135.4478) -> (-2.2324, 132.8399)
  line L49 (-2.2324, 132.8399) -> (-1.4531, 132.7271)
  spline S146 degree 3 poles (-0.7114, 133.0929) (-0.8481, 133.0748) (-1.1356, 133.0369) (-1.3438, 132.8337) (-1.4531, 132.7271) knots 0 0 0 0 0.040273 0.0847 0.0847 0.0847 0.0847
  spline S147 degree 3 poles (-0.173, 132.8621) (-0.2482, 132.9294) (-0.4015, 133.0666) (-0.6067, 133.084) (-0.7114, 133.0929) knots 0 0 0 0 0.029423 0.060008 0.060008 0.060008 0.060008
  spline S148 degree 3 poles (0.0338, 132.17) (0.0296, 132.3088) (0.022, 132.5592) (-0.1129, 132.7687) (-0.173, 132.8621) knots 0 0 0 0 0.040704 0.073449 0.073449 0.073449 0.073449
  spline S149 degree 3 poles (-0.1747, 131.4334) (-0.1141, 131.533) (0.0228, 131.7579) (0.0299, 132.0225) (0.0338, 132.17) knots 0 0 0 0 0.034394 0.077732 0.077732 0.077732 0.077732
  spline S150 degree 3 poles (-0.684, 131.189) (-0.587, 131.2) (-0.3891, 131.2223) (-0.2471, 131.3622) (-0.1747, 131.4334) knots 0 0 0 0 0.028435 0.057968 0.057968 0.057968 0.057968
  spline S151 degree 3 poles (-1.1489, 131.3787) (-1.0797, 131.3234) (-0.9433, 131.2143) (-0.7696, 131.1974) (-0.684, 131.189) knots 0 0 0 0 0.025952 0.051182 0.051182 0.051182 0.051182
  spline S152 degree 3 poles (-1.3915, 131.8931) (-1.3728, 131.7921) (-1.337, 131.5989) (-1.2096, 131.4499) (-1.1489, 131.3787) knots 0 0 0 0 0.030207 0.057777 0.057777 0.057777 0.057777
  line L50 (-1.3915, 131.8931) -> (-2.3486, 131.794)
  spline S153 degree 3 poles (-1.8256, 130.7926) (-1.9571, 130.9302) (-2.2276, 131.2131) (-2.3075, 131.5969) (-2.3486, 131.794) knots 0 0 0 0 0.055929 0.115014 0.115014 0.115014 0.115014
  line L51 (-4.2695, 131.2266) -> (-4.2695, 132.5289)
  line L52 (-4.2695, 132.5289) -> (-2.9535, 132.5289)
  line L53 (-2.9535, 132.5289) -> (-2.9535, 133.4278)
  line L54 (-2.9535, 133.4278) -> (-4.2695, 133.4278)
  line L55 (-4.2695, 133.4278) -> (-4.2695, 134.7301)
  line L56 (-4.2695, 134.7301) -> (-5.1445, 134.7301)
  line L57 (-5.1445, 134.7301) -> (-5.1445, 133.4278)
  line L58 (-5.1445, 133.4278) -> (-6.457, 133.4278)
  line L59 (-6.457, 133.4278) -> (-6.457, 132.5289)
  line L60 (-6.457, 132.5289) -> (-5.1445, 132.5289)
  line L61 (-5.1445, 132.5289) -> (-5.1445, 131.2266)
  line L62 (-5.1445, 131.2266) -> (-4.2695, 131.2266)
  line L63 (-13.3696, 130.42) -> (-11.5752, 135.4307)
  line L64 (-11.5752, 135.4307) -> (-12.6484, 135.4307)
  line L65 (-12.6484, 135.4307) -> (-13.8755, 131.7222)
  line L66 (-13.8755, 131.7222) -> (-15.1436, 135.4307)
  line L67 (-15.1436, 135.4307) -> (-16.2407, 135.4307)
  line L68 (-16.2407, 135.4307) -> (-14.4497, 130.42)
  line L69 (-14.4497, 130.42) -> (-13.3696, 130.42)
  spline S154 degree 3 poles (-18.3001, 131.5787) (-18.3379, 131.5346) (-18.41, 131.4505) (-18.4687, 131.3567) (-18.4966, 131.3121) knots 0 0 0 0 0.017402 0.033163 0.033163 0.033163 0.033163
  spline S155 degree 3 poles (-17.7241, 132.1324) (-17.8494, 132.0183) (-18.0463, 131.8388) (-18.2323, 131.6481) (-18.3001, 131.5787) knots 0 0 0 0 0.050814 0.079907 0.079907 0.079907 0.079907
  spline S156 degree 3 poles (-17.0952, 132.7716) (-17.1754, 132.68) (-17.3726, 132.4549) (-17.5932, 132.2525) (-17.7241, 132.1324) knots 0 0 0 0 0.036482 0.089726 0.089726 0.089726 0.089726
  spline S157 degree 3 poles (-16.7107, 133.4124) (-16.7596, 133.306) (-16.8643, 133.0785) (-17.015, 132.8782) (-17.0952, 132.7716) knots 0 0 0 0 0.035023 0.074928 0.074928 0.074928 0.074928
  spline S158 degree 3 poles (-16.5894, 134.0567) (-16.5943, 133.9456) (-16.604, 133.7251) (-16.6753, 133.5162) (-16.7107, 133.4124) knots 0 0 0 0 0.033165 0.06586 0.06586 0.06586 0.06586
  spline S159 degree 3 poles (-17.0132, 135.0513) (-16.8896, 134.9094) (-16.6409, 134.6237) (-16.6066, 134.2465) (-16.5894, 134.0567) knots 0 0 0 0 0.054981 0.110602 0.110602 0.110602 0.110602
  spline S160 degree 3 poles (-18.1787, 135.4513) (-17.9503, 135.4395) (-17.5219, 135.4175) (-17.175, 135.1678) (-17.0132, 135.0513) knots 0 0 0 0 0.066973 0.125562 0.125562 0.125562 0.125562
  spline S161 degree 3 poles (-19.3067, 135.106) (-19.142, 135.2067) (-18.7963, 135.4179) (-18.391, 135.4398) (-18.1787, 135.4513) knots 0 0 0 0 0.056979 0.119613 0.119613 0.119613 0.119613
  spline S162 degree 3 poles (-19.8433, 133.9679) (-19.8079, 134.2065) (-19.7432, 134.6426) (-19.4427, 134.9616) (-19.3067, 135.106) knots 0 0 0 0 0.070363 0.128535 0.128535 0.128535 0.128535
  line L70 (-19.8433, 133.9679) -> (-18.8862, 133.8721)
  spline S163 degree 3 poles (-18.6812, 134.4737) (-18.7344, 134.3958) (-18.8576, 134.2155) (-18.8759, 133.9965) (-18.8862, 133.8721) knots 0 0 0 0 0.027875 0.064515 0.064515 0.064515 0.064515
  spline S164 degree 3 poles (-18.2026, 134.6549) (-18.2962, 134.6489) (-18.4748, 134.6374) (-18.6146, 134.5265) (-18.6812, 134.4737) knots 0 0 0 0 0.027379 0.052265 0.052265 0.052265 0.052265
  spline S165 degree 3 poles (-17.7258, 134.4823) (-17.7917, 134.5325) (-17.9319, 134.6397) (-18.1088, 134.6496) (-18.2026, 134.6549) knots 0 0 0 0 0.024288 0.051759 0.051759 0.051759 0.051759
  spline S166 degree 3 poles (-17.5532, 133.9884) (-17.5579, 134.0866) (-17.5667, 134.2692) (-17.6756, 134.4149) (-17.7258, 134.4823) knots 0 0 0 0 0.028738 0.053388 0.053388 0.053388 0.053388
  spline S167 degree 3 poles (-17.7515, 133.4005) (-17.6937, 133.4963) (-17.5842, 133.678) (-17.5632, 133.8888) (-17.5532, 133.9884) knots 0 0 0 0 0.033093 0.062734 0.062734 0.062734 0.062734
  spline S168 degree 3 poles (-18.5479, 132.5802) (-18.3685, 132.7449) (-18.0872, 133.0032) (-17.8408, 133.2948) (-17.7515, 133.4005) knots 0 0 0 0 0.072938 0.114424 0.114424 0.114424 0.114424
  spline S169 degree 3 poles (-19.6279, 131.3787) (-19.4967, 131.5582) (-19.1775, 131.9945) (-18.7812, 132.3631) (-18.5479, 132.5802) knots 0 0 0 0 0.066554 0.16187 0.16187 0.16187 0.16187
  spline S170 degree 3 poles (-19.9561, 130.42) (-19.9283, 130.5872) (-19.8721, 130.9249) (-19.7099, 131.2264) (-19.6279, 131.3787) knots 0 0 0 0 0.050461 0.101951 0.101951 0.101951 0.101951
  line L71 (-19.9561, 130.42) -> (-16.5894, 130.42)
  line L72 (-16.5894, 130.42) -> (-16.5894, 131.3121)
  line L73 (-16.5894, 131.3121) -> (-18.4966, 131.3121)
  line L74 (-21.2686, 135.4513) -> (-22.0479, 135.4513)
  spline S171 degree 3 poles (-22.6528, 134.6497) (-22.5185, 134.766) (-22.2594, 134.9903) (-22.1166, 135.3014) (-22.0479, 135.4513) knots 0 0 0 0 0.052597 0.101463 0.101463 0.101463 0.101463
  spline S172 degree 3 poles (-23.4697, 134.1832) (-23.3363, 134.2377) (-23.0438, 134.3572) (-22.7905, 134.5467) (-22.6528, 134.6497) knots 0 0 0 0 0.043078 0.094413 0.094413 0.094413 0.094413
  line L75 (-23.4697, 134.1832) -> (-23.4697, 133.3116)
  spline S173 degree 3 poles (-22.229, 134.0396) (-22.4136, 133.8858) (-22.7869, 133.5747) (-23.2405, 133.4) (-23.4697, 133.3116) knots 0 0 0 0 0.071555 0.144721 0.144721 0.144721 0.144721
  line L76 (-22.229, 134.0396) -> (-22.229, 130.42)
  line L77 (-22.229, 130.42) -> (-21.2686, 130.42)
  line L78 (-21.2686, 130.42) -> (-21.2686, 135.4513)
  line L79 (-25.6333, 131.1412) -> (-25.6333, 132.4434)
  line L80 (-25.6333, 132.4434) -> (-24.3174, 132.4434)
  line L81 (-24.3174, 132.4434) -> (-24.3174, 133.3424)
  line L82 (-24.3174, 133.3424) -> (-25.6333, 133.3424)
  line L83 (-25.6333, 133.3424) -> (-25.6333, 134.6446)
  line L84 (-25.6333, 134.6446) -> (-26.5083, 134.6446)
  line L85 (-26.5083, 134.6446) -> (-26.5083, 133.3424)
  line L86 (-26.5083, 133.3424) -> (-27.8208, 133.3424)
  line L87 (-27.8208, 133.3424) -> (-27.8208, 132.4434)
  line L88 (-27.8208, 132.4434) -> (-26.5083, 132.4434)
  line L89 (-26.5083, 132.4434) -> (-26.5083, 131.1412)
  line L90 (-26.5083, 131.1412) -> (-25.6333, 131.1412)
  line L91 (-24.798, 113.7564) -> (-24.798, 114.7169)
  line L92 (-24.798, 114.7169) -> (-26.6847, 114.7169)
  line L93 (-26.6847, 114.7169) -> (-26.6847, 113.7564)
  line L94 (-26.6847, 113.7564) -> (-24.798, 113.7564)
  line L95 (-21.9919, 117.4513) -> (-22.7712, 117.4513)
  spline S174 degree 3 poles (-23.3762, 116.6497) (-23.2418, 116.766) (-22.9827, 116.9903) (-22.8399, 117.3014) (-22.7712, 117.4513) knots 0 0 0 0 0.052597 0.101463 0.101463 0.101463 0.101463
  spline S175 degree 3 poles (-24.193, 116.1832) (-24.0596, 116.2377) (-23.7671, 116.3572) (-23.5138, 116.5467) (-23.3762, 116.6497) knots 0 0 0 0 0.043078 0.094413 0.094413 0.094413 0.094413
  line L96 (-24.193, 116.1832) -> (-24.193, 115.3116)
  spline S176 degree 3 poles (-22.9523, 116.0396) (-23.1369, 115.8858) (-23.5102, 115.5747) (-23.9638, 115.4) (-24.193, 115.3116) knots 0 0 0 0 0.071555 0.144721 0.144721 0.144721 0.144721
  line L97 (-22.9523, 116.0396) -> (-22.9523, 112.42)
  line L98 (-22.9523, 112.42) -> (-21.9919, 112.42)
  line L99 (-21.9919, 112.42) -> (-21.9919, 117.4513)
  spline S177 degree 3 poles (-19.0234, 113.5787) (-19.0612, 113.5346) (-19.1333, 113.4505) (-19.192, 113.3567) (-19.2199, 113.3121) knots 0 0 0 0 0.017402 0.033163 0.033163 0.033163 0.033163
  spline S178 degree 3 poles (-18.4474, 114.1324) (-18.5727, 114.0183) (-18.7696, 113.8388) (-18.9556, 113.6481) (-19.0234, 113.5787) knots 0 0 0 0 0.050814 0.079907 0.079907 0.079907 0.079907
  spline S179 degree 3 poles (-17.8185, 114.7716) (-17.8987, 114.68) (-18.0959, 114.4549) (-18.3165, 114.2525) (-18.4474, 114.1324) knots 0 0 0 0 0.036482 0.089726 0.089726 0.089726 0.089726
  spline S180 degree 3 poles (-17.434, 115.4124) (-17.4829, 115.306) (-17.5876, 115.0785) (-17.7383, 114.8782) (-17.8185, 114.7716) knots 0 0 0 0 0.035023 0.074928 0.074928 0.074928 0.074928
  spline S181 degree 3 poles (-17.3127, 116.0567) (-17.3176, 115.9456) (-17.3273, 115.7251) (-17.3986, 115.5162) (-17.434, 115.4124) knots 0 0 0 0 0.033165 0.06586 0.06586 0.06586 0.06586
  spline S182 degree 3 poles (-17.7365, 117.0513) (-17.6129, 116.9094) (-17.3642, 116.6237) (-17.3299, 116.2465) (-17.3127, 116.0567) knots 0 0 0 0 0.054981 0.110602 0.110602 0.110602 0.110602
  spline S183 degree 3 poles (-18.902, 117.4513) (-18.6736, 117.4395) (-18.2452, 117.4175) (-17.8984, 117.1678) (-17.7365, 117.0513) knots 0 0 0 0 0.066974 0.125562 0.125562 0.125562 0.125562
  spline S184 degree 3 poles (-20.03, 117.106) (-19.8653, 117.2067) (-19.5196, 117.4179) (-19.1143, 117.4398) (-18.902, 117.4513) knots 0 0 0 0 0.056979 0.119613 0.119613 0.119613 0.119613
  spline S185 degree 3 poles (-20.5666, 115.9679) (-20.5312, 116.2065) (-20.4665, 116.6426) (-20.166, 116.9616) (-20.03, 117.106) knots 0 0 0 0 0.070363 0.128535 0.128535 0.128535 0.128535
  line L100 (-20.5666, 115.9679) -> (-19.6095, 115.8721)
  spline S186 degree 3 poles (-19.4045, 116.4737) (-19.4577, 116.3958) (-19.581, 116.2155) (-19.5992, 115.9965) (-19.6095, 115.8721) knots 0 0 0 0 0.027875 0.064515 0.064515 0.064515 0.064515
  spline S187 degree 3 poles (-18.926, 116.6549) (-19.0195, 116.6489) (-19.1981, 116.6374) (-19.3379, 116.5265) (-19.4045, 116.4737) knots 0 0 0 0 0.027379 0.052265 0.052265 0.052265 0.052265
  spline S188 degree 3 poles (-18.4491, 116.4823) (-18.515, 116.5325) (-18.6552, 116.6397) (-18.8321, 116.6496) (-18.926, 116.6549) knots 0 0 0 0 0.024288 0.051759 0.051759 0.051759 0.051759
  spline S189 degree 3 poles (-18.2765, 115.9884) (-18.2813, 116.0866) (-18.29, 116.2692) (-18.3989, 116.4149) (-18.4491, 116.4823) knots 0 0 0 0 0.028738 0.053388 0.053388 0.053388 0.053388
  spline S190 degree 3 poles (-18.4748, 115.4005) (-18.417, 115.4963) (-18.3075, 115.678) (-18.2865, 115.8888) (-18.2765, 115.9884) knots 0 0 0 0 0.033093 0.062734 0.062734 0.062734 0.062734
  spline S191 degree 3 poles (-19.2712, 114.5802) (-19.0918, 114.7449) (-18.8105, 115.0032) (-18.5641, 115.2948) (-18.4748, 115.4005) knots 0 0 0 0 0.072938 0.114424 0.114424 0.114424 0.114424
  spline S192 degree 3 poles (-20.3512, 113.3787) (-20.22, 113.5582) (-19.9008, 113.9945) (-19.5045, 114.3631) (-19.2712, 114.5802) knots 0 0 0 0 0.066554 0.16187 0.16187 0.16187 0.16187
  spline S193 degree 3 poles (-20.6794, 112.42) (-20.6516, 112.5872) (-20.5954, 112.9249) (-20.4332, 113.2264) (-20.3512, 113.3787) knots 0 0 0 0 0.050461 0.101951 0.101951 0.101951 0.101951
  line L101 (-20.6794, 112.42) -> (-17.3127, 112.42)
  line L102 (-17.3127, 112.42) -> (-17.3127, 113.3121)
  line L103 (-17.3127, 113.3121) -> (-19.2199, 113.3121)
  line L104 (-14.0929, 112.42) -> (-12.2985, 117.4307)
  line L105 (-12.2985, 117.4307) -> (-13.3718, 117.4307)
  line L106 (-13.3718, 117.4307) -> (-14.5988, 113.7222)
  line L107 (-14.5988, 113.7222) -> (-15.8669, 117.4307)
  line L108 (-15.8669, 117.4307) -> (-16.964, 117.4307)
  line L109 (-16.964, 117.4307) -> (-15.173, 112.42)
  line L110 (-15.173, 112.42) -> (-14.0929, 112.42)
  spline S194 degree 3 poles (6.7442, 112.42) (6.5301, 112.4338) (6.1173, 112.4603) (5.7791, 112.6973) (5.6163, 112.8114) knots 0 0 0 0 0.062972 0.121456 0.121456 0.121456 0.121456
  spline S195 degree 3 poles (7.9439, 112.8848) (7.7712, 112.7493) (7.4189, 112.4728) (6.972, 112.4378) (6.7442, 112.42) knots 0 0 0 0 0.064351 0.13125 0.13125 0.13125 0.13125
  spline S196 degree 3 poles (8.4258, 114.0094) (8.4054, 113.7973) (8.3644, 113.3713) (8.0845, 113.0474) (7.9439, 112.8848) knots 0 0 0 0 0.062273 0.125073 0.125073 0.125073 0.125073
  spline S197 degree 3 poles (8.1678, 114.7852) (8.243, 114.6707) (8.3977, 114.4352) (8.4163, 114.1538) (8.4258, 114.0094) knots 0 0 0 0 0.040399 0.083017 0.083017 0.083017 0.083017
  spline S198 degree 3 poles (7.4791, 115.1988) (7.6146, 115.1595) (7.8809, 115.0823) (8.0733, 114.8831) (8.1678, 114.7852) knots 0 0 0 0 0.041536 0.081592 0.081592 0.081592 0.081592
  spline S199 degree 3 poles (8.2002, 116.2515) (8.1628, 116.039) (8.0826, 115.583) (7.6891, 115.3325) (7.4791, 115.1988) knots 0 0 0 0 0.061982 0.132968 0.132968 0.132968 0.132968
  spline S200 degree 3 poles (7.8482, 117.0855) (7.9509, 116.9606) (8.151, 116.717) (8.1841, 116.404) (8.2002, 116.2515) knots 0 0 0 0 0.047352 0.092313 0.092313 0.092313 0.092313
  spline S201 degree 3 poles (6.7134, 117.5367) (6.9347, 117.5208) (7.3617, 117.4902) (7.69, 117.2171) (7.8482, 117.0855) knots 0 0 0 0 0.064735 0.124887 0.124887 0.124887 0.124887
  spline S202 degree 3 poles (5.9666, 117.3812) (6.083, 117.4265) (6.3231, 117.5201) (6.5807, 117.531) (6.7134, 117.5367) knots 0 0 0 0 0.037209 0.07675 0.07675 0.07675 0.07675
  spline S203 degree 3 poles (5.4471, 116.9539) (5.5168, 117.0404) (5.6605, 117.2184) (5.8626, 117.3259) (5.9666, 117.3812) knots 0 0 0 0 0.032959 0.067885 0.067885 0.067885 0.067885
  spline S204 degree 3 poles (5.1685, 116.2276) (5.2, 116.3667) (5.258, 116.6225) (5.3878, 116.8501) (5.4471, 116.9539) knots 0 0 0 0 0.042495 0.07817 0.07817 0.07817 0.07817
  line L111 (5.1685, 116.2276) -> (6.0538, 116.0772)
  spline S205 degree 3 poles (6.2657, 116.5763) (6.2129, 116.5089) (6.098, 116.3621) (6.0693, 116.1772) (6.0538, 116.0772) knots 0 0 0 0 0.025264 0.055024 0.055024 0.055024 0.055024
  spline S206 degree 3 poles (6.6861, 116.7471) (6.6071, 116.7401) (6.4495, 116.726) (6.3269, 116.6261) (6.2657, 116.5763) knots 0 0 0 0 0.023211 0.046318 0.046318 0.046318 0.046318
  spline S207 degree 3 poles (7.086, 116.5968) (7.03, 116.6406) (6.9128, 116.7324) (6.7639, 116.7421) (6.6861, 116.7471) knots 0 0 0 0 0.020834 0.04362 0.04362 0.04362 0.04362
  spline S208 degree 3 poles (7.2364, 116.1934) (7.2314, 116.2721) (7.222, 116.4222) (7.1298, 116.5405) (7.086, 116.5968) knots 0 0 0 0 0.023038 0.043945 0.043945 0.043945 0.043945
  spline S209 degree 3 poles (7.0313, 115.7166) (7.0911, 115.7825) (7.2138, 115.9178) (7.2287, 116.1) (7.2364, 116.1934) knots 0 0 0 0 0.025943 0.053218 0.053218 0.053218 0.053218
  spline S210 degree 3 poles (6.4366, 115.5474) (6.5545, 115.5485) (6.7693, 115.5505) (6.9499, 115.665) (7.0313, 115.7166) knots 0 0 0 0 0.034551 0.062931 0.062931 0.062931 0.062931
  line L112 (6.4366, 115.5474) -> (6.3306, 114.7647)
  spline S211 degree 3 poles (6.7715, 114.8365) (6.7037, 114.8326) (6.5544, 114.8239) (6.4096, 114.7856) (6.3306, 114.7647) knots 0 0 0 0 0.020331 0.044771 0.044771 0.044771 0.044771
  spline S212 degree 3 poles (7.2466, 114.6246) (7.1785, 114.6864) (7.0432, 114.8091) (6.8616, 114.8274) (6.7715, 114.8365) knots 0 0 0 0 0.026832 0.05326 0.05326 0.05326 0.05326
  spline S213 degree 3 poles (7.4415, 114.0504) (7.4356, 114.1623) (7.4246, 114.3727) (7.3034, 114.5443) (7.2466, 114.6246) knots 0 0 0 0 0.032834 0.061749 0.061749 0.061749 0.061749
  spline S214 degree 3 poles (7.2381, 113.442) (7.2973, 113.5273) (7.4239, 113.7097) (7.4354, 113.9321) (7.4415, 114.0504) knots 0 0 0 0 0.030567 0.065292 0.065292 0.065292 0.065292
  spline S215 degree 3 poles (6.7374, 113.2164) (6.8328, 113.226) (7.0247, 113.2454) (7.1667, 113.3762) (7.2381, 113.442) knots 0 0 0 0 0.027961 0.056262 0.056262 0.056262 0.056262
  spline S216 degree 3 poles (6.2657, 113.4044) (6.3343, 113.3495) (6.4725, 113.2392) (6.6487, 113.224) (6.7374, 113.2164) knots 0 0 0 0 0.025738 0.0518 0.0518 0.0518 0.0518
  spline S217 degree 3 poles (6.0264, 113.9478) (6.0447, 113.8392) (6.0787, 113.6372) (6.2066, 113.4779) (6.2657, 113.4044) knots 0 0 0 0 0.032415 0.060264 0.060264 0.060264 0.060264
  line L113 (6.0264, 113.9478) -> (5.0967, 113.835)
  spline S218 degree 3 poles (5.6163, 112.8114) (5.4825, 112.9538) (5.2098, 113.244) (5.1349, 113.6356) (5.0967, 113.835) knots 0 0 0 0 0.057366 0.116928 0.116928 0.116928 0.116928
  line L114 (3.0323, 112.5054) -> (4.8267, 117.5162)
  line L115 (4.8267, 117.5162) -> (3.7535, 117.5162)
  line L116 (3.7535, 117.5162) -> (2.5264, 113.8077)
  line L117 (2.5264, 113.8077) -> (1.2583, 117.5162)
  line L118 (1.2583, 117.5162) -> (0.1612, 117.5162)
  line L119 (0.1612, 117.5162) -> (1.9522, 112.5054)
  line L120 (1.9522, 112.5054) -> (3.0323, 112.5054)
  spline S219 degree 3 poles (-1.8178, 112.42) (-2.0319, 112.4338) (-2.4447, 112.4603) (-2.7829, 112.6973) (-2.9458, 112.8114) knots 0 0 0 0 0.062972 0.121456 0.121456 0.121456 0.121456
  spline S220 degree 3 poles (-0.6181, 112.8848) (-0.7908, 112.7493) (-1.1431, 112.4728) (-1.59, 112.4378) (-1.8178, 112.42) knots 0 0 0 0 0.064351 0.13125 0.13125 0.13125 0.13125
  spline S221 degree 3 poles (-0.1362, 114.0094) (-0.1566, 113.7973) (-0.1976, 113.3713) (-0.4776, 113.0474) (-0.6181, 112.8848) knots 0 0 0 0 0.062273 0.125073 0.125073 0.125073 0.125073
  spline S222 degree 3 poles (-0.3942, 114.7852) (-0.319, 114.6707) (-0.1644, 114.4352) (-0.1457, 114.1538) (-0.1362, 114.0094) knots 0 0 0 0 0.040399 0.083017 0.083017 0.083017 0.083017
  spline S223 degree 3 poles (-1.083, 115.1988) (-0.9474, 115.1595) (-0.6811, 115.0823) (-0.4887, 114.8831) (-0.3942, 114.7852) knots 0 0 0 0 0.041536 0.081592 0.081592 0.081592 0.081592
  spline S224 degree 3 poles (-0.3618, 116.2515) (-0.3992, 116.039) (-0.4794, 115.583) (-0.8729, 115.3325) (-1.083, 115.1988) knots 0 0 0 0 0.061982 0.132968 0.132968 0.132968 0.132968
  spline S225 degree 3 poles (-0.7138, 117.0855) (-0.6112, 116.9606) (-0.411, 116.717) (-0.3779, 116.404) (-0.3618, 116.2515) knots 0 0 0 0 0.047352 0.092313 0.092313 0.092313 0.092313
  spline S226 degree 3 poles (-1.8486, 117.5367) (-1.6273, 117.5208) (-1.2003, 117.4902) (-0.872, 117.2171) (-0.7138, 117.0855) knots 0 0 0 0 0.064735 0.124887 0.124887 0.124887 0.124887
  spline S227 degree 3 poles (-2.5954, 117.3812) (-2.479, 117.4265) (-2.2389, 117.5201) (-1.9813, 117.531) (-1.8486, 117.5367) knots 0 0 0 0 0.037209 0.07675 0.07675 0.07675 0.07675